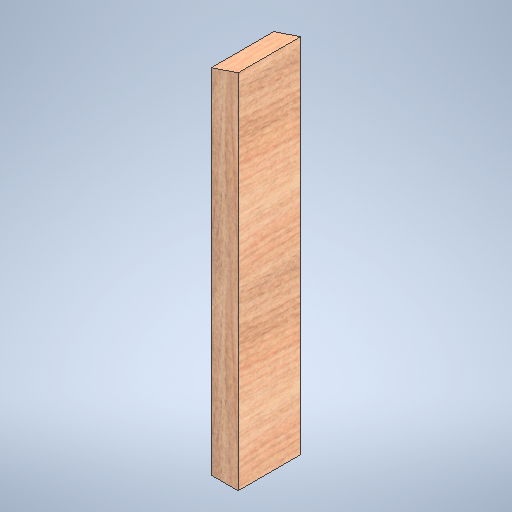
# Autodesk Inventor part: Stud_Between_Top_Plate_And_Rafter_4
Saved by Autodesk Inventor 2025 (Build 290162010, 162A)
## iProperties
Created: 2024-09-30
Part Number: Stud_Between_Top_Plate_And_Rafter_4
Material: Wood (Birch)
Document SubType Name: Modeling
Designer: Tom
Density: 0.55 g/cm^3
Appearance: Birch - Natural Polished
Author: Tom
Autodesk Inventor part; units mm, degrees
ref_plane "YZ Plane" through (0, 0, 0) normal (1, 0, 0) x (0, 1, 0)
ref_plane "XZ Plane" through (0, 0, 0) normal (0, 1, 0) x (-1, 0, 0)
ref_plane "XY Plane" through (0, 0, 0) normal (0, 0, 1) x (1, 0, 0)
sketch "Sketch1" plane through (0, 0, 0) normal (0, 0, 1) x (1, 0, 0)
  line L0 (0, 0) -> (38.1, 0)
  line L1 (38.1, 0) -> (38.1, 514.858)
  line L2 (38.1, 514.858) -> (0, 502.1326)
  line L3 (0, 502.1326) -> (0, 0)
  dimension "d2" = 38.1
  dimension "d5" = 502.1326
  dimension "d6" = 514.858
  constraints: 8 end point, 1 horizontal, 1 parallel, 1 perpendicular
  measures "d2" distance between parallel lines of L1 L3
  measures "d5" distance of L2.end L0.start
  measures "d6" distance of L0.end L1.end
extrude "Extrusion1" add sketch "Sketch1" along normal blind 88.9
body "Solid1"
